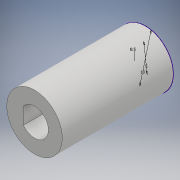
# Autodesk Inventor part: motor-gear-base
Saved by Autodesk Inventor 2017 (Build 210142000, 142)
## iProperties
Created: 2026-03-25
Part Number: motor-gear-base
Material: Generic
Document SubType Name: Modeling
Designer: a
Density: 1 g/cm^3
Appearance: Default
Author: a
Autodesk Inventor part; units mm, degrees
ref_plane "YZ Plane" through (0, 0, 0) normal (1, 0, 0) x (0, 1, 0)
ref_plane "XZ Plane" through (0, 0, 0) normal (0, 1, 0) x (-1, 0, 0)
ref_plane "XY Plane" through (0, 0, 0) normal (0, 0, 1) x (1, 0, 0)
sketch "Sketch1" plane through (0, 0, 0) normal (0, 1, 0) x (-1, 0, 0)
  circle A0 centre (0, 0) radius 2.5
  line L0 (2, 1.5) -> (2, -1.5)
  circle A1 centre (0, 0) radius 5
  dimension "d0" = 5
  dimension "d1" = 0.5
  dimension "d2" = 10
  constraints: 2 centre point, 2 coincident, 2 end point, 2 point on circle, 1 vertical
  measures "d0" diameter of A0
  measures "d1" distance edge to line of A0 L0
  measures "d2" diameter of A1
extrude "Extrusion1" add sketch "Sketch1" against normal blind 20 contours A0 L0 | A1 picked at (2.0912, -0.3466)
extrude "Extrusion2" add sketch "Sketch1" against normal blind 2 contours L0 A0 picked at (0.2258, 0.7583)
body "Solid1"
